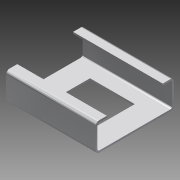
# Autodesk Inventor part: YagiFanMetal
Saved by Autodesk Inventor 2014 (Build 180170000, 170)
## iProperties
Created: 2015-04-30
Part Number: YagiFanMetal
Material: Generic
Document SubType Name: Sheet Metal
Designer: Owner
Density: 1 g/cm^3
Sheet Metal Rule: Default
Appearance: Aluminum - Polished
Author: Owner
Autodesk Inventor part; units mm, degrees
ref_plane "YZ Plane" through (0, 0, 0) normal (1, 0, 0) x (0, 1, 0)
ref_plane "XZ Plane" through (0, 0, 0) normal (0, 1, 0) x (-1, 0, 0)
ref_plane "XY Plane" through (0, 0, 0) normal (0, 0, 1) x (1, 0, 0)
sketch "Sketch1" plane through (0, 0, 0) normal (0, 1, 0) x (-1, 0, 0)
  line L0 (-44.9038, 48.5577) -> (35.0962, 48.5577)
  line L1 (35.0962, 48.5577) -> (35.0962, -21.2923)
  line L2 (35.0962, -21.2923) -> (-44.9038, -21.2923)
  line L3 (-44.9038, -21.2923) -> (-44.9038, 48.5577)
  line L4 (-24.9038, 33.6327) -> (15.0962, 33.6327)
  line L5 (15.0962, 33.6327) -> (15.0962, -6.3673)
  line L6 (15.0962, -6.3673) -> (-24.9038, -6.3673)
  line L7 (-24.9038, -6.3673) -> (-24.9038, 33.6327)
  point P0 (0, 0)
  dimension "d0" = 80
  dimension "d1" = 69.85
  dimension "d23" = 40
  dimension "d24" = 40
  dimension "d25" = 20
  dimension "d26" = 14.925
  measures "d0" distance of L0.start L0.end
  measures "d1" distance of L0.end L1.end
  measures "d23" distance of L4.start L4.end
  measures "d24" distance of L4.end L5.end
  measures "d25" distance between parallel lines of L3 L7
  measures "d26" distance between parallel lines of L0 L4
extrude "Plate1" add sketch "Sketch1" along normal blind 1.5875
sketch "Sketch2" plane through (44.9038, 0, 46.9702) normal (0, 0, 1) x (1, 0, 0)
  line L0 (-80, 0) -> (0, 0)
  line L1 (0, 0) -> (0, 25)
  line L2 (0, 25) -> (-80, 25)
  line L3 (-80, 25) -> (-80, 0)
  constraints: 6 end point, 1 horizontal, 1 perpendicular, 1 vertical
edge flange "Flange1" height 25 angle 90 thickness 1.5875 bend radius 1.5875 thickness toward (0, 0, 1) relief straight relief width 1.5875 relief depth 0.7937 edges at (4.9038, 1.5875, 48.5577) wall of the first edge with corners at (-35.0962, 0, 46.9702) (44.9038, 0, 46.9702) (44.9038, 25, 46.9702) (-35.0962, 25, 46.9702)
bend "Bend1"
corner "Corner1"
sketch "Sketch3" plane through (-35.0962, 0, -19.7048) normal (0, 0, -1) x (-1, 0, 0)
  line L0 (-80, 0) -> (0, 0)
  line L1 (0, 0) -> (0, 25)
  line L2 (0, 25) -> (-80, 25)
  line L3 (-80, 25) -> (-80, 0)
  constraints: 6 end point, 1 horizontal, 1 perpendicular, 1 vertical
edge flange "Flange2" height 25 angle 90 thickness 1.5875 bend radius 1.5875 thickness toward (0, 0, -1) relief straight relief width 1.5875 relief depth 0.7937 edges at (4.9038, 1.5875, -21.2923) wall of the first edge with corners at (44.9038, 0, -19.7048) (-35.0962, 0, -19.7048) (-35.0962, 25, -19.7048) (44.9038, 25, -19.7048)
bend "Bend2"
corner "Corner2"
sketch "Sketch6" plane through (-35.0962, 23.4125, -21.2923) normal (0, 1, 0) x (-1, 0, 0)
  line L0 (-80, 0) -> (0, 0)
  line L1 (0, 0) -> (0, 10)
  line L2 (0, 10) -> (-80, 10)
  line L3 (-80, 10) -> (-80, 0)
  constraints: 6 end point, 1 horizontal, 1 perpendicular, 1 vertical
edge flange "Flange3" height 10 angle 90 thickness 1.5875 bend radius 1.5875 thickness toward (0, 1, 0) relief straight relief width 1.5875 relief depth 0.7937 edges at (4.9038, 25, -19.7048) wall of the first edge with corners at (44.9038, 23.4125, -21.2923) (-35.0962, 23.4125, -21.2923) (-35.0962, 23.4125, -11.2923) (44.9038, 23.4125, -11.2923)
bend "Bend3"
corner "Corner3"
sketch "Sketch7" plane through (44.9038, 23.4125, 48.5577) normal (0, 1, 0) x (-1, 0, 0)
  line L0 (80, 0) -> (0, 0)
  line L1 (0, 0) -> (0, -10)
  line L2 (0, -10) -> (80, -10)
  line L3 (80, -10) -> (80, 0)
  constraints: 6 end point, 1 horizontal, 1 perpendicular, 1 vertical
edge flange "Flange4" height 10 angle 90 thickness 1.5875 bend radius 1.5875 thickness toward (0, 1, 0) relief straight relief width 1.5875 relief depth 0.7937 edges at (4.9038, 25, 46.9702) wall of the first edge with corners at (-35.0962, 23.4125, 48.5577) (44.9038, 23.4125, 48.5577) (44.9038, 23.4125, 38.5577) (-35.0962, 23.4125, 38.5577)
bend "Bend4"
corner "Corner4"
equation "\"d3\" = BendReliefWidth"
equation "\"d4\" = BendReliefDepth"
equation "\"d5\" = MinimumRemnant"
equation "\"d6\" = BendRadius"
equation "\"d9\" = BendRadius"
equation "\"d10\" = CornerReliefSize"
equation "\"d11\" = GapSize"
equation "\"d12\" = JacobiRadiusSize"
equation "\"d13\" = BendReliefWidth"
equation "\"d14\" = BendReliefDepth"
equation "\"d15\" = MinimumRemnant"
equation "\"d16\" = BendRadius"
equation "\"d19\" = BendRadius"
equation "\"d20\" = CornerReliefSize"
equation "\"d21\" = GapSize"
equation "\"d22\" = JacobiRadiusSize"
equation "\"d27\" = BendReliefWidth"
equation "\"d28\" = BendReliefDepth"
equation "\"d29\" = MinimumRemnant"
equation "\"d30\" = BendRadius"
equation "\"d33\" = BendRadius"
equation "\"d34\" = CornerReliefSize"
equation "\"d35\" = GapSize"
equation "\"d36\" = JacobiRadiusSize"
equation "\"d37\" = BendReliefWidth"
equation "\"d38\" = BendReliefDepth"
equation "\"d39\" = MinimumRemnant"
equation "\"d40\" = BendRadius"
equation "\"d43\" = BendRadius"
equation "\"d44\" = CornerReliefSize"
equation "\"d45\" = GapSize"
equation "\"d46\" = JacobiRadiusSize"
equation "\"BendRadius\" = Thickness"
equation "\"BendReliefWidth\" = Thickness"
equation "\"BendReliefDepth\" = 0.5 * Thickness"
equation "\"CornerReliefSize\" = 4 * Thickness"
equation "\"MinimumRemnant\" = 2 * Thickness"
equation "\"TransitionRadius\" = BendRadius"
equation "\"JacobiRadiusSize\" = BendRadius"
equation "\"GapSize\" = Thickness"
equation "\"d2\" = BendRadius"
equation "\"Thickness\" = 1.5875"
body "Solid1"
